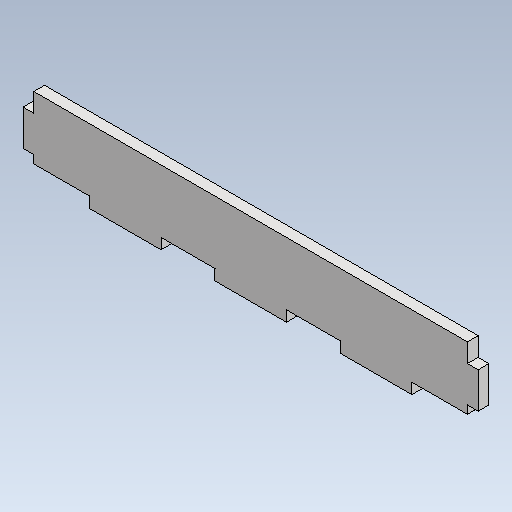
# Autodesk Inventor part: bed_acrylic_upper_front
Saved by Autodesk Inventor 2025 (Build 290162000, 162)
## iProperties
Created: 2025-08-24
Part Number: bed_acrylic_upper_front
Material: Generic
Document SubType Name: Modeling
Designer: HP
Density: 1 g/cm^3
Appearance: Default
Author: HP
Autodesk Inventor part; units mm, degrees
ref_plane "YZ Plane" through (0, 0, 0) normal (1, 0, 0) x (0, 1, 0)
ref_plane "XZ Plane" through (0, 0, 0) normal (0, 1, 0) x (-1, 0, 0)
ref_plane "XY Plane" through (0, 0, 0) normal (0, 0, 1) x (1, 0, 0)
sketch "Sketch1" plane through (0, 0, 0) normal (0, 0, 1) x (1, 0, 0)
  line L0 (-63.5, -10.25) -> (63.5, -10.25)
  line L1 (63.5, -10.25) -> (63.5, 10.25)
  line L2 (63.5, 10.25) -> (-63.5, 10.25)
  line L3 (-63.5, 10.25) -> (-63.5, -10.25)
  line L4 (-63.5, -10.25) -> (63.5, 10.25) construction
  line L5 (63.5, -10.25) -> (-63.5, 10.25) construction
  line L6 (-63.5, -5) -> (-60.5, -5)
  line L7 (-60.5, -5) -> (-60.5, 5) construction
  line L8 (-60.5, 5) -> (-63.5, 5)
  line L9 (-63.5, 5) -> (-63.5, -5)
  line L10 (-63.5, -5) -> (-60.5, 5) construction
  line L11 (-60.5, -5) -> (-63.5, 5) construction
  line L12 (-45, -10.25) -> (-25, -10.25)
  line L13 (-25, -10.25) -> (-25, -7.25)
  line L14 (-25, -7.25) -> (-45, -7.25) construction
  line L15 (-45, -7.25) -> (-45, -10.25)
  line L16 (-45, -10.25) -> (-25, -7.25) construction
  line L17 (-25, -10.25) -> (-45, -7.25) construction
  line L18 (-10, -10.25) -> (10, -10.25)
  line L19 (10, -10.25) -> (10, -7.25)
  line L20 (10, -7.25) -> (-10, -7.25) construction
  line L21 (-10, -7.25) -> (-10, -10.25)
  line L22 (-10, -10.25) -> (10, -7.25) construction
  line L23 (10, -10.25) -> (-10, -7.25) construction
  line L24 (25, -7.25) -> (25, -10.25)
  line L25 (45, -10.25) -> (45, -7.25)
  line L26 (25, -10.25) -> (45, -10.25)
  line L27 (45, -10.25) -> (25, -7.25) construction
  line L28 (45, -7.25) -> (25, -7.25) construction
  line L29 (25, -10.25) -> (45, -7.25) construction
  line L30 (-45, -7.25) -> (-63.5, -7.25)
  line L31 (-25, -7.25) -> (-10, -7.25)
  line L32 (10, -7.25) -> (25, -7.25)
  line L33 (45, -7.25) -> (63.5, -7.25)
  line L34 (-60.5, 5) -> (-60.5, 10.25)
  line L35 (-60.5, -5) -> (-60.5, -10.25)
  point P0 (0, 0)
  point P1 (-62, 0)
  point P2 (-63.5, 0)
  point P3 (-35, -8.75)
  point P4 (0, -8.75)
  point P5 (35, -8.75)
  point P6 (0, -10.25)
  point P7 (-45, -10.25)
  point P8 (-25, -10.25)
  point P9 (-10, -10.25)
  point P10 (10, -10.25)
  point P11 (25, -10.25)
  point P12 (45, -10.25)
  point P13 (-60.5, -7.25)
  dimension "d0" = 20.5
  dimension "d1" = 127
  dimension "d2" = 10
  dimension "d3" = 3
  dimension "d4" = 3
  dimension "d5" = 20
  dimension "d6" = 3
  dimension "d7" = 20
  dimension "d8" = 35
  dimension "d9" = 3
  dimension "d10" = 20
  dimension "d11" = 35
  constraints: 72 end point, 12 midpoint, 10 parallel, 7 perpendicular, 6 point on line, 5 horizontal, 4 collinear, 1 horizontal alignment, 1 vertical alignment
  measures "d0" distance between parallel lines of L0 L2
  measures "d1" distance between parallel lines of L1 L3
  measures "d2" distance between parallel lines of L6 L8
  measures "d3" distance between parallel lines of L7 L9
  measures "d4" distance between parallel lines of L12 L14
  measures "d5" distance between parallel lines of L13 L15
  measures "d6" distance between parallel lines of L18 L20
  measures "d7" distance between parallel lines of L19 L21
  measures "d8" distance of point (0, -8.75) point (-35, -8.75)
  measures "d9" distance between parallel lines of L26 L28
  measures "d10" distance between parallel lines of L25 L24
  measures "d11" distance of point (35, -8.75) point (0, -8.75)
extrude "Extrusion1" add sketch "Sketch1" along normal blind 3 contours L3 L6 L35 L30 | L15 L30 L35 L6 L3 L8 L34 L2 L1 L33 L25 L0 L24 L32 L19 L21 L31 L13 | L3 L2 L34 L8
extrude "Extrusion2" cut sketch "Sketch1" along normal through all contours L3 L30 L35 L0 | L35 L30 L15 L0 | L3 L6 L35 L30 | L13 L31 L21 L0 | L3 L2 L34 L8 | L19 L32 L24 L0 | L25 L33 L1 L0
mirror "Mirror1" about plane through (0, 0, 0) normal (1, 0, 0) of "Extrusion2"
equation "\"d4\" = d3"
equation "\"d6\" = d3"
equation "\"d7\" = d5"
equation "\"d9\" = d6"
equation "\"d10\" = d7"
equation "\"d11\" = d8"
body "Solid1"
